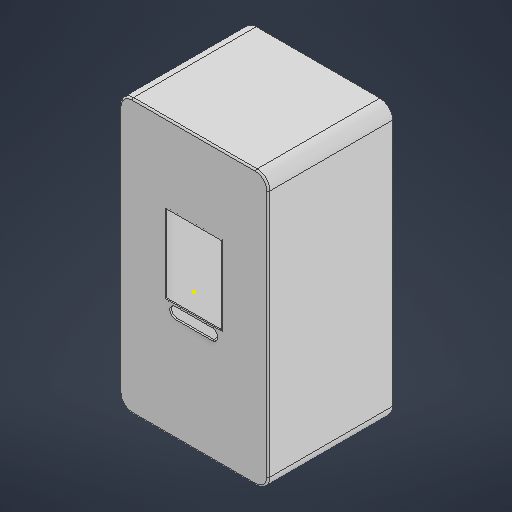
# Autodesk Inventor part: MainBody
Saved by Autodesk Inventor 2026.2 (Build 302298010, 298A)
## iProperties
Created: 2026-03-28
Part Number: MainBody
Material: Generic
Document SubType Name: Modeling
Designer: tp2105
Density: 1 g/cm^3
Appearance: Default
Author: tp2105
Autodesk Inventor part; units mm, degrees
ref_plane "YZ Plane" through (0, 0, 0) normal (1, 0, 0) x (0, 1, 0)
ref_plane "XZ Plane" through (0, 0, 0) normal (0, 1, 0) x (-1, 0, 0)
ref_plane "XY Plane" through (0, 0, 0) normal (0, 0, 1) x (1, 0, 0)
sketch "Sketch1" plane through (0, 0, 0) normal (0, 0, 1) x (1, 0, 0)
  line L0 (0, 0) -> (100, 0) construction
  line L1 (-60, -110) -> (60, -110)
  line L2 (60, -110) -> (60, 110)
  line L3 (60, 110) -> (-60, 110)
  line L4 (-60, 110) -> (-60, -110)
  line L5 (-60, -110) -> (60, 110) construction
  line L6 (60, -110) -> (-60, 110) construction
  dimension "d5" = 120
  dimension "d6" = 220
  constraints: 14 end point, 2 horizontal, 2 midpoint, 2 parallel, 1 perpendicular
  measures "d5" distance of L3.end L2.end
  measures "d6" distance of L2.end L1.end
extrude "Extrusion1" add sketch "Sketch1" along normal mid plane 100
fillet "Fillet1" radius 10.25 4 edges at (60, 110, 0) (-60, 110, 0) (60, -110, 0) (-60, -110, 0)
fillet "Fillet2" radius 1.25 8 edges at (-56.9978, 106.9978, 50) (-60, 0, 50) (-56.9978, -106.9978, 50) (0, -110, 50) (56.9978, -106.9978, 50) (60, 0, 50) (56.9978, 106.9978, 50) (0, 110, 50)
sketch "Sketch3" plane through (0, 0, 50) normal (0, 0, 1) x (1, 0, 0)
  line L0 (-22.64, 46.3465) -> (21.36, 46.3465)
  line L1 (21.36, 46.3465) -> (21.36, -15.6535)
  line L2 (21.36, -15.6535) -> (-22.64, -15.6535)
  line L3 (-22.64, -15.6535) -> (-22.64, 46.3465)
  line L4 (-22.64, 46.3465) -> (21.36, -15.6535) construction
  line L5 (21.36, 46.3465) -> (-22.64, -15.6535) construction
  point P0 (0, 0)
  point P1 (-0.64, 15.3465)
  dimension "d21" = 44
  dimension "d22" = 62
  constraints: 12 end point, 2 midpoint, 2 parallel, 1 horizontal, 1 perpendicular
  measures "d21" distance of L1.end L2.end
  measures "d22" distance of L0.end L1.end
extrude "Extrusion3" cut sketch "Sketch3" against normal blind 0.5
shell "Shell2" thickness 1.5 removed faces 2 at (-7.9733, 25.6799, 49.5) at (-20, 33.25, -50)
fillet "Fillet4" radius 0.5 4 edges at (-22.64, 15.3465, 50) (-0.64, 46.3465, 50) (21.36, 15.3465, 50) (-0.64, -15.6535, 50)
sketch "Sketch4" plane through (0, 0, 50) normal (0, 0, 1) x (1, 0, 0)
  line L0 (-23.14, -16.1535) -> (21.86, -16.1535) projected
  line L1 (21.86, -16.1535) -> (2.86, -16.1535)
  line L2 (21.86, -16.1535) -> (15.86, -16.1535)
  circle A0 centre (10.86, -22.1535) radius 4
  circle A1 centre (-6.64, -22.1535) radius 2
  line L3 (21.36, -15.6535) -> (-22.64, -15.6535) projected
  line L4 (21.36, -15.6535) -> (14.36, -15.6535)
  circle A2 centre (-6.64, -22.1535) radius 3
  line L5 (-14.86, -22.1535) -> (14.86, -22.1535) construction
  line L6 (-14.86, -26.6535) -> (14.86, -26.6535)
  line L7 (14.86, -17.6535) -> (-14.86, -17.6535)
  arc A3 (-14.86, -17.6535) -> (-14.86, -26.6535) centre (-14.86, -22.1535) ccw
  arc A4 (14.86, -26.6535) -> (14.86, -17.6535) centre (14.86, -22.1535) ccw
  point P0 (0, 0)
  point P1 (0, -22.1535)
  dimension "d33" = 4
  dimension "d35" = 6
  dimension "d36" = 9
  constraints: 14 end point, 4 centre point, 4 point on circle, 4 tangent, 3 point on line, 1 coincident, 1 horizontal, 1 horizontal alignment, 1 midpoint, 1 parallel, 2 other
  measures "d33" diameter of A1
  measures "d35" diameter of A2
  measures "d36" diameter of A4
extrude "Extrusion4" cut sketch "Sketch4" against normal blind 4 contours A0 | A1 | A2 | A3 L7 A4 L6
sketch "Sketch5" plane through (0, 0, 50) normal (0, 0, 1) x (1, 0, 0)
  point P0 (0, 0)
body "Solid1"
